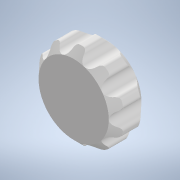
# Autodesk Inventor part: Колпачок
Saved by Autodesk Inventor 2020 (Build 240168000, 168)
## iProperties
Created: 2020-12-08
Part Number: Колпачок
Material: Типовые
Document SubType Name: Modeling
Designer: User
Density: 1 g/cm^3
Appearance: По умолчанию
Author: User
Autodesk Inventor part; units mm, degrees
ref_plane "YZ Plane" through (0, 0, 0) normal (1, 0, 0) x (0, 1, 0)
ref_plane "XZ Plane" through (0, 0, 0) normal (0, 1, 0) x (-1, 0, 0)
ref_plane "XY Plane" through (0, 0, 0) normal (0, 0, 1) x (1, 0, 0)
sketch "Эскиз1" plane through (0, 0, 0) normal (0, 0, 1) x (1, 0, 0)
  line L0 (-3.5, 0) -> (-3.5, 2.0207) projected
  line L1 (-3.5, -2.0207) -> (-3.5, 0) projected
  line L2 (-3.5, 2.0207) -> (-1.75, 3.0311) projected
  line L3 (-1.75, 3.0311) -> (0, 4.0415) projected
  line L4 (0, 4.0415) -> (1.75, 3.0311) projected
  line L5 (1.75, 3.0311) -> (3.5, 2.0207) projected
  line L6 (3.5, 2.0207) -> (3.5, 0) projected
  line L7 (3.5, 0) -> (3.5, -2.0207) projected
  line L8 (3.5, -2.0207) -> (1.75, -3.0311) projected
  line L9 (1.75, -3.0311) -> (0, -4.0415) projected
  line L10 (0, -4.0415) -> (-1.75, -3.0311) projected
  line L11 (-1.75, -3.0311) -> (-3.5, -2.0207) projected
  circle A0 centre (0, 0) radius 11
  dimension "d0" = 22
  constraints: 1 centre point, 1 coincident
  measures "d0" diameter of A0
ref_plane "РабПлоскость1" through (-20, -130.8333, -3.37) normal (0, 0, 1) x (1, 0, 0)
extrude "Выдавливание1" add sketch "Эскиз1" against normal up to surface (3.37 mm away)
sketch "Эскиз2" plane through (0, 0, 0) normal (0, 0, 1) x (1, 0, 0)
  circle A0 centre (0, 0) radius 11 projected
extrude "Выдавливание2" add sketch "Эскиз2" along normal blind 5
chamfer "Фаска1" distance 2 angle 45 2 edges at (-11, 0, -3.37) (-11, 0, 5)
sketch "Эскиз3" plane through (0, 0, 5) normal (0, 0, 1) x (1, 0, 0)
  circle A0 centre (0, 0) radius 11 construction
  circle A1 centre (0, 0) radius 11 construction
  circle A2 centre (-11, 0) radius 2
  circle A3 centre (-8.8992, -6.4656) radius 2
  circle A4 centre (-3.3992, -10.4616) radius 2
  circle A5 centre (3.3992, -10.4616) radius 2
  circle A6 centre (8.8992, -6.4656) radius 2
  circle A7 centre (11, 0) radius 2
  circle A8 centre (8.8992, 6.4656) radius 2
  circle A9 centre (3.3992, 10.4616) radius 2
  circle A10 centre (-3.3992, 10.4616) radius 2
  circle A11 centre (-8.8992, 6.4656) radius 2
  dimension "d8" = 4
  dimension "d9" = 22
  dimension "d10" = 11
  dimension "d13" = 360
  constraints: 10 centre point, 1 horizontal alignment, 22 other
  measures "d8" diameter of A2
  measures "d9" diameter of A0
  measures "d10" distance of point (0, 0) A2.centre
extrude "Выдавливание3" cut sketch "Эскиз3" against normal through all
fillet "Сопряжение1" radius 1 20 edges at (-10.8182, 1.9917, 0.815) (-9.9228, 4.7474, 0.815) (-10.8182, -1.9917, 0.815) (-9.9228, -4.7474, 0.815) (-7.5814, 7.9701, 0.815) (-5.2372, 9.6732, 0.815) (-7.5814, -7.9701, 0.815) (-1.4488, 10.9042, 0.815) (1.4488, 10.9042, 0.815) (5.2372, 9.6732, 0.815) (7.5814, 7.9701, 0.815) (9.9228, 4.7474, 0.815) (10.8182, 1.9917, 0.815) (10.8182, -1.9917, 0.815) (9.9228, -4.7474, 0.815) (7.5814, -7.9701, 0.815) (-5.2372, -9.6732, 0.815) (-1.4488, -10.9042, 0.815) (1.4488, -10.9042, 0.815) (5.2372, -9.6732, 0.815)
equation "\"d10\" = 0.5 * d9"
